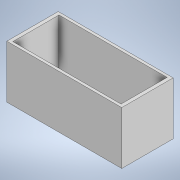
# Autodesk Inventor part: BatteryHolder
Saved by Autodesk Inventor 2022 (Build 260153000, 153)
## iProperties
Created: 2022-02-22
Part Number: BatteryHolder
Material: Generic
Document SubType Name: Modeling
Designer: merky
Density: 1 g/cm^3
Appearance: Default
Author: merky
Autodesk Inventor part; units mm, degrees
ref_plane "YZ Plane" through (0, 0, 0) normal (1, 0, 0) x (0, 1, 0)
ref_plane "XZ Plane" through (0, 0, 0) normal (0, 1, 0) x (-1, 0, 0)
ref_plane "XY Plane" through (0, 0, 0) normal (0, 0, 1) x (1, 0, 0)
sketch "Sketch1" plane through (0, 0, 0) normal (0, 1, 0) x (-1, 0, 0)
  line L0 (-90.805, 38.735) -> (90.805, 38.735)
  line L1 (90.805, 38.735) -> (90.805, -38.735)
  line L2 (90.805, -38.735) -> (-90.805, -38.735)
  line L3 (-90.805, -38.735) -> (-90.805, 38.735)
  line L4 (-90.805, 38.735) -> (90.805, -38.735) construction
  line L5 (90.805, 38.735) -> (-90.805, -38.735) construction
  line L6 (96.52, 43.18) -> (-96.52, 43.18)
  line L7 (-96.52, 43.18) -> (-96.52, -43.18)
  line L8 (-96.52, -43.18) -> (96.52, -43.18)
  line L9 (96.52, -43.18) -> (96.52, 43.18)
  line L10 (96.52, 43.18) -> (-96.52, -43.18) construction
  line L11 (-96.52, 43.18) -> (96.52, -43.18) construction
  point P0 (0, 0)
  dimension "d0" = 181.61
  dimension "d1" = 77.47
  dimension "d2" = 193.04
  dimension "d3" = 86.36
  constraints: 24 end point, 4 midpoint, 4 parallel, 2 horizontal, 2 perpendicular
  measures "d0" distance of L1.end L2.end
  measures "d1" distance of L0.end L1.end
  measures "d2" distance of L8.end L7.end
  measures "d3" distance of L7.end L6.end
extrude "Extrusion1" add sketch "Sketch1" against normal blind 5.08 contours L0 L1 L2 L3 | L9 L8 L7 L6
extrude "Extrusion2" add sketch "Sketch1" along normal blind 83.566
body "Solid1"
